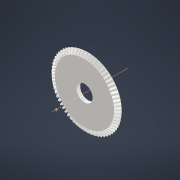
# Autodesk Inventor part: Bevel Gear1
Saved by Autodesk Inventor 2022 (Build 260153000, 153)
## iProperties
CustomPartVersion: 1
Created: 2021-09-10
Part Number: Bevel Gear1
Material: Steel, Mild
Document SubType Name: Modeling
Designer: Andres
Categories: <?xml version="1.0" encoding="UTF-16"?> <MemberInstance><Categories><FamilyTemplate><FamilyTemplateParameter ValueType="xs:double" Id="1" ObjectReferenceKey="da_z" ObjectType="kUserParameterObject"/><FamilyTemplateParameter ValueType="xs:double" Id="2" ObjectReferenceKey="da_b" ObjectType="kUserParameterObject"/><FamilyTemplateParameter ValueType="xs:double" Id="3" ObjectReferenceKey="da_beta" ObjectType="kUserParameterObject"/><FamilyTemplateParameter ValueType="xs:double" Id="4" ObjectReferenceKey="da_dae" ObjectType="kUserParameterObject"/><FamilyTemplateParameter ValueType="xs:double" Id="5" ObjectReferenceKey="da_ve" ObjectType="kUserParameterObject"/><FamilyTemplateParameter ValueType="xs:double" Id="6" ObjectReferenceKey="da_omega" ObjectType="kUserParameterObject"/><FamilyTemplateParameter ValueType="xs:string" Id="7" ObjectReferenceKey="EAIAABAAAAAAHwAAAAAAAIAAAAAAAAAA" ObjectType="83914240" SubObjectId="SurfaceGeometry"/></FamilyTemplate><ParamToTemplateMap><ParamToTemplate CategoryParameter="//CategoryParameter[@InternalName='046C89C9-8512-4d59-83FE-43B91F4F132A']" TemplateParameter="1"/><ParamToTemplate CategoryParameter="//CategoryParameter[@InternalName='2552DF32-E462-4b46-AEBF-C6C7768E72AC']" TemplateParameter="2"/><ParamToTemplate CategoryParameter="//CategoryParameter[@InternalName='C9EE641D-15FC-4fae-A226-E94C4372FDD7']" TemplateParameter="3"/><ParamToTemplate><ParamToTemplate CategoryParameter="//CategoryParameter[@InternalName='00B6519A-459B-49c7-AD84-2E56D39A5744']" ConstantValue="0.000000"/></ParamToTemplate><ParamToTemplate><ParamToTemplate CategoryParameter="//CategoryParameter[@InternalName='04B31F0E-C7A6-4894-AA32-9629BEFACF47']" ConstantValue="1.000000"/></ParamToTemplate><ParamToTemplate><ParamToTemplate CategoryParameter="//CategoryParameter[@InternalName='43CBEC2E-7847-49e7-A936-2F7889FCB2D9']" ConstantValue="0.200000"/></ParamToTemplate><ParamToTemplate><ParamToTemplate CategoryParameter="//CategoryParameter[@InternalName='B1EFC894-105D-4ebd-86BF-FA20ED196853']" ConstantValue="0.300000"/></ParamToTemplate><ParamToTemplate><ParamToTemplate CategoryParameter="//CategoryParameter[@InternalName='51175063-3D10-4879-93E8-6246FE8B403D']" ConstantValue="2060000000.000000"/></ParamToTemplate><ParamToTemplate><ParamToTemplate CategoryParameter="//CategoryParameter[@InternalName='A3A52E27-4454-46a9-B0BD-C932399B70AF']" ConstantValue="0.300000"/></ParamToTemplate><ParamToTemplate CategoryParameter="//CategoryParameter[@InternalName='2A200944-5A8C-41ca-B96E-8520D2E510F1']" TemplateParameter="4"/><ParamToTemplate><ParamToTemplate CategoryParameter="//CategoryParameter[@InternalName='1A637F62-92C8-44bc-B81F-10802510B579']" ConstantValue="11.541463"/></ParamToTemplate><ParamToTemplate CategoryParameter="//CategoryParameter[@InternalName='B52DD4BE-6863-48fb-BF58-89EF6F9EC65C']" TemplateParameter="5"/><ParamToTemplate><ParamToTemplate CategoryParameter="//CategoryParameter[@InternalName='3956BFF2-84D2-457d-93C2-9B0613DEBA67']" ConstantValue="4.902986"/></ParamToTemplate><ParamToTemplate CategoryParameter="//CategoryParameter[@InternalName='739CFA02-461B-4bf8-8049-181FCAD8B28F']" TemplateParameter="6"/><ParamToTemplate><ParamToTemplate CategoryParameter="//CategoryParameter[@InternalName='A27E999F-E2CE-4481-8A2A-EBF499C4C3C5']" ConstantValue="0.000000"/></ParamToTemplate><ParamToTemplate><ParamToTemplate CategoryParameter="//CategoryParameter[@InternalName='9E1B4470-B2D3-4ff1-B813-535BB4CDF51A']" ConstantValue="3520000.000000"/></ParamToTemplate><ParamToTemplate><ParamToTemplate CategoryParameter="//CategoryParameter[@InternalName='F8452263-BFF6-458c-9FB1-07C4B99E95CD']" ConstantValue="11400000.000000"/></ParamToTemplate><ParamToTemplate><ParamToTemplate CategoryParameter="//CategoryParameter[@InternalName='3E3BB259-FD49-497f-8171-6EBC954A3479']" ConstantValue="2.000000"/></ParamToTemplate><ParamToTemplate CategoryParameter="//CategoryParameter[@InternalName='27C3BAF2-7550-4e4b-AE2C-0DB134B7D9B7']" TemplateParameter="7"/></ParamToTemplateMap><Category DisplayName="Gear" InternalName="DC85795E-93AB-48d5-8EEE-5A27447B64BD" Mnemonic="Gear"><CategoryParameter DisplayName="z" InternalName="046C89C9-8512-4d59-83FE-43B91F4F132A" Mnemonic="z"/><CategoryParameter DisplayName="b" InternalName="2552DF32-E462-4b46-AEBF-C6C7768E72AC" Mnemonic="b"/><CategoryParameter DisplayName="||b|" InternalName="C9EE641D-15FC-4fae-A226-E94C4372FDD7" Mnemonic="beta"/><CategoryParameter DisplayName="x" InternalName="00B6519A-459B-49c7-AD84-2E56D39A5744" Mnemonic="x"/><CategoryParameter DisplayName="a*" InternalName="04B31F0E-C7A6-4894-AA32-9629BEFACF47" Mnemonic="a"/><CategoryParameter DisplayName="c*" InternalName="43CBEC2E-7847-49e7-A936-2F7889FCB2D9" Mnemonic="c"/><CategoryParameter DisplayName="r|.f|*" InternalName="B1EFC894-105D-4ebd-86BF-FA20ED196853" Mnemonic="rf"/><CategoryParameter DisplayName="E" InternalName="51175063-3D10-4879-93E8-6246FE8B403D" Mnemonic="E"/><CategoryParameter DisplayName="||m|" InternalName="A3A52E27-4454-46a9-B0BD-C932399B70AF" Mnemonic="mi"/><Category DisplayName="BevelGear" InternalName="0C98F69A-0C2B-4791-B2FE-7691BB227E77" Mnemonic="BevelGear"><CategoryParameter DisplayName="d|.ae|" InternalName="2A200944-5A8C-41ca-B96E-8520D2E510F1" Mnemonic="dae"/><CategoryParameter DisplayName="d|.ai|" InternalName="1A637F62-92C8-44bc-B81F-10802510B579" Mnemonic="dai"/><CategoryParameter DisplayName="A|.e|" InternalName="B52DD4BE-6863-48fb-BF58-89EF6F9EC65C" Mnemonic="ve"/><CategoryParameter DisplayName="A|.i|" InternalName="3956BFF2-84D2-457d-93C2-9B0613DEBA67" Mnemonic="vi"/><CategoryParameter DisplayName="||S|" InternalName="739CFA02-461B-4bf8-8049-181FCAD8B28F" Mnemonic="omega"/><CategoryParameter DisplayName="x|.t|" InternalName="A27E999F-E2CE-4481-8A2A-EBF499C4C3C5" Mnemonic="xt"/><CategoryParameter DisplayName="||s||.Flim|" InternalName="9E1B4470-B2D3-4ff1-B813-535BB4CDF51A" Mnemonic="sFlim"/><CategoryParameter DisplayName="||s||.Hlim|" InternalName="F8452263-BFF6-458c-9FB1-07C4B99E95CD" Mnemonic="sHlim"/><CategoryParameter DisplayName="type" InternalName="3E3BB259-FD49-497f-8171-6EBC954A3479" Mnemonic="type"/><CategoryParameter DisplayName="PitchDiameter" InternalName="27C3BAF2-7550-4e4b-AE2C-0DB134B7D9B7" Mnemonic="IDS_PITCHDIAM"/></Category></Category></Categories></MemberInstance>
Mass: 60.9118 g
Surface Area: 34.3074 cm^2
Volume: 7.7496 cm^3
Density: 7.86 g/cm^3
Appearance: Steel
Author: Andres
Autodesk Inventor part; units mm, degrees
ref_plane "XZ Plane" through (0, 0, 0) normal (0, 1, 0) x (-1, 0, 0)
ref_plane "Mesh Plane2" through (0, 0, 0) normal (0.9987955, 0.0490677, 0) x (0, 0, 1)
sketch "Teeth Body Sketch" plane through (0, 0, 0) normal (1, 0, 0) x (0, 1, 0)
  line L0 (0, 0) -> (62.4038, -58.7922) construction
  line L1 (62.4038, -58.7922) -> (65.3302, -55.5065)
  line L2 (65.3302, -55.5065) -> (0, 0) construction
  line L3 (64, -57) -> (0, 0) construction
  line L4 (55.1224, -51.9322) -> (57.7073, -49.0299)
  line L5 (62.4038, -58.7922) -> (55.1224, -51.9322)
  line L6 (65.3302, -55.5065) -> (57.7073, -49.0299)
  line L7 (0, -70.488) -> (0, 11.748) projected
  line L8 (0, -57) -> (65.3302, -57) construction
  dimension "d0" = 128
  dimension "d1" = 124.8076
  dimension "d2" = 130.6603
  dimension "d3" = 10
  dimension "d4" = 55.5065
  constraints: 16 end point, 4 point on line, 3 perpendicular, 2 collinear, 1 horizontal alignment, 1 vertical alignment
  measures "d0" diameter of L3.start L7
  measures "d1" diameter of L0.end L7
  measures "d2" diameter of L1.end L7
  measures "d3" distance between parallel lines of L1 L4
  measures "d4" vertical distance of L1.end L0.start
revolve "Teeth Body" add sketch "Teeth Body Sketch" angle 360 about axis through (0, 0, 0) along (0, 0, 1)
ref_plane "Tooth Plane" through (0, 64, -57) normal (0, -0.7467652, 0.6650878) x (1, 0, 0)
sketch "Start Sketch" plane through (0, 64, -57) normal (0, -0.7467652, 0.6650878) x (1, 0, 0)
  line L0 (0, -105.204) -> (0, 21.4234) projected
  arc A0 (-0.6566, -2.928) -> (-3.0101, 3.2745) centre (-33.1011, -11.6912) ccw
  arc A1 (3.0101, 3.2745) -> (0.6566, -2.928) centre (33.1011, -11.6912) ccw
  line L1 (-0.6566, -2.928) -> (0.6566, -2.928)
  arc A2 (3.0101, 3.2745) -> (-3.0101, 3.2745) centre (0, -96.2279) ccw
  dimension "d7" = 33.6071
  dimension "d8" = 33.1011
  dimension "d9" = 84.5367
  dimension "d57" = 99.5479
  dimension "d58" = 93.2999
  constraints: 6 point on circle, 3 centre point, 3 symmetric about line, 2 end point, 1 coincident, 1 perpendicular, 1 other
  measures "d7" radius of A0
  measures "d8" horizontal distance of point (0, -96.228) A0.centre
  measures "d9" vertical distance of point (0, -96.228) A0.centre
  measures "d57" radius of A2
  measures "d58" distance from line of A2.centre L1
sketch "End Sketch" plane through (0, 56.3681, -50.2028) normal (0, -0.7467652, 0.6650878) x (1, 0, 0)
  line L0 (0, -92.2122) -> (0, 18.7778) projected
  arc A0 (-0.5783, -2.5788) -> (-2.6511, 2.884) centre (-29.1538, -10.297) ccw
  arc A1 (2.6511, 2.884) -> (0.5783, -2.5788) centre (29.1538, -10.297) ccw
  line L1 (-0.5783, -2.5788) -> (0.5783, -2.5788)
  arc A2 (2.6511, 2.884) -> (-2.6511, 2.884) centre (0, -84.7528) ccw
  dimension "d12" = 29.5995
  dimension "d15" = 29.1538
  dimension "d16" = 74.4558
  dimension "d59" = 87.6769
  dimension "d60" = 82.174
  constraints: 6 point on circle, 3 centre point, 3 symmetric about line, 2 end point, 1 coincident, 1 other
  measures "d12" radius of A0
  measures "d15" horizontal distance of A0.centre point (0, -84.753)
  measures "d16" vertical distance of A0.centre point (0, -84.753)
  measures "d59" radius of A2
  measures "d60" distance from line of A2.centre L1
loft "Loft" cut profiles "Start Sketch", "End Sketch"
pattern_circular "Circular Pattern" count 64 over 360 about axis through (0, 0, 0) along (0, 0, 1) of "Loft"
ref_plane "End Plane" through (0, 56.3681, -50.2028) normal (0, -0.7467652, 0.6650878) x (1, 0, 0)
sketch3d "3D Sketch Right"
ref_plane "End Plane Right" through (-3.5891, 56.2537, -50.2028) normal (0.0475486, -0.7452499, 0.6650878) x (0.9979708, 0.0636728, 0)
sketch "End Sketch Right" plane through (-3.5891, 56.2537, -50.2028) normal (0.0475486, -0.7452499, 0.6650878) x (0.9979708, 0.0636728, 0)
  arc A0 (-0.5783, -2.5788) -> (-2.6511, 2.884) centre (-29.1538, -10.297) ccw
  line L0 (0, -105.4152) -> (0, 23.5844) projected
  arc A1 (2.6511, 2.884) -> (0.5783, -2.5788) centre (29.1538, -10.297) ccw
  line L1 (-0.5783, -2.5788) -> (0.5783, -2.5788)
  arc A2 (2.6511, 2.884) -> (-2.6511, 2.884) centre (0, -84.7528) ccw
  dimension "d70" = 29.1538
  dimension "d71" = 74.4558
  dimension "d72" = 29.5995
  dimension "d73" = 82.174
  dimension "d74" = 87.6769
  constraints: 6 point on circle, 3 centre point, 3 symmetric about line, 2 end point, 1 coincident, 1 perpendicular, 1 other
  measures "d70" horizontal distance of A2.centre A0.centre
  measures "d71" vertical distance of point (0, -84.753) A0.centre
  measures "d72" radius of A0
  measures "d73" distance from line of point (0, -84.753) L1
  measures "d74" radius of A2
feature "Loft Right" [suppressed]
pattern_circular "Circular Pattern Right" [suppressed]
sketch3d "3D Sketch Left"
ref_plane "End Plane Left" through (3.5913, 56.2537, -50.2039) normal (-0.0475768, -0.7452413, 0.6650953) x (0.9979684, -0.0637111, 0)
sketch "End Sketch Left" plane through (3.5913, 56.2537, -50.2039) normal (-0.0475768, -0.7452413, 0.6650953) x (0.9979684, -0.0637111, 0)
  line L0 (0, -108.6763) -> (0, 26.8468) projected
  arc A0 (-0.5783, -2.5781) -> (-2.6511, 2.8848) centre (-29.1538, -10.2962) ccw
  arc A1 (2.6511, 2.8848) -> (0.5783, -2.5781) centre (29.1538, -10.2962) ccw
  line L1 (-0.5783, -2.5781) -> (0.5783, -2.5781)
  ellipse E0 centre (0, -36.6135) end of major axis (57.7073, -36.6135) minor radius 38.3809 projected
  arc A2 (2.6511, 2.8848) -> (-2.6511, 2.8848) centre (0, -84.7521) ccw
  dimension "d56" = 38.3809
  dimension "d30" = 29.5995
  dimension "d31" = 29.1538
  dimension "d32" = 74.4558
  dimension "d61" = 87.6769
  dimension "d62" = 82.174
  constraints: 6 point on circle, 3 centre point, 3 symmetric about line, 2 end point, 1 coincident, 2 other
  measures "d30" radius of A0
  measures "d31" horizontal distance of point (0, -84.752) A0.centre
  measures "d32" vertical distance of A0.centre point (0, -84.752)
  measures "d61" radius of A2
  measures "d62" distance from line of point (0, -84.752) L1
feature "Loft Left" [suppressed]
pattern_circular "Circular Pattern Left" [suppressed]
sketch "Body Sketch" plane through (0, 0, 0) normal (1, 0, 0) x (0, 1, 0)
  line L0 (0, -60.1595) -> (0, -50.2227) projected
  line L1 (62.4038, -58.7922) -> (55.1224, -51.9322) projected
  line L2 (55.1224, -51.9322) -> (0, -51.9322)
  line L3 (62.4038, -58.7922) -> (0, -58.7922)
  constraints: 4 end point, 2 perpendicular, 2 point on line
revolve "Fix Body" add sketch "Body Sketch" angle 360 about axis through (0, 0, 0) along (0, 0, 1)
sketch "Sketch6" plane through (0, 0, 0) normal (1, 0, 0) x (0, 1, 0)
  line L0 (64, -57) -> (0, 0) projected
  line L1 (0, -68.4) -> (0, 11.4) projected
surface revolve "Pitch Diameter" sketch "Sketch6" angle 360 about axis through (0, 0, 0) along (0, 0, 1) shown no curves L0
sketch "Sketch8" plane through (0, 0, -58.7922) normal (0, 0, -1) x (-0.9986295, 0.052336, 0)
  circle A0 centre (0, 0) radius 15
  dimension "d94" = 30
  constraints: 1 centre point, 1 coincident
  measures "d94" diameter of A0
extrude "Extrusion1" cut sketch "Sketch8" against normal through all
equation "\"d0\" = da_de"
equation "\"d1\" = da_dfe"
equation "\"d2\" = da_dae"
equation "\"d3\" = da_b"
equation "\"d4\" = da_ve"
equation "\"d7\" = fd_rr"
equation "\"d8\" = fd_x"
equation "\"d9\" = fd_y"
equation "\"d57\" = 0.5 * fd_dva + 0.3 * da_he"
equation "\"d58\" = 0.5 * fd_dva - 1.12 * da_he"
equation "\"da_teethtype\" = 0"
equation "\"da_b\" = 10"
equation "\"da_de\" = 128"
equation "\"da_dae\" = 130.66035"
equation "\"da_dfe\" = 124.80758"
equation "\"da_le\" = 85.70298"
equation "\"da_omega\" = 90deg"
equation "\"da_beta\" = 0"
equation "\"da_delta\" = 48.310942deg"
equation "\"da_alpha\" = 20deg"
equation "\"da_he\" = 4.4"
equation "\"da_ve\" = 55.50647"
equation "\"da_zv\" = 96.227902"
equation "\"fd_loft\" = da_b + 0.05 * da_he"
equation "\"fd_x\" = fd_x1 + fd_x2"
equation "\"fd_y\" = fd_y1 - fd_y2"
equation "\"fd_dd\" = fd_dva - 0.8 * da_he"
equation "\"da_dvw\" = 192.4558"
equation "\"d11\" = fd_loft"
equation "\"da_dm\" = 120.53235"
equation "\"da_x\" = 0"
equation "\"da_m\" = 2"
equation "\"d50\" = da_omega"
equation "\"fd_rr\" = 33.607126"
equation "\"fd_dva\" = 196.455804"
equation "\"fd_x1\" = 1.588178"
equation "\"fd_x2\" = 31.512887"
equation "\"fd_y1\" = 96.214795"
equation "\"fd_y2\" = 11.678049"
body "Solid1"
body "Srf1"
